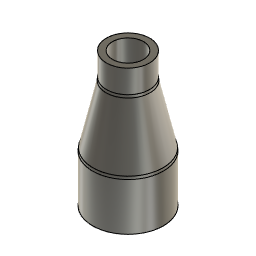
v1.0.0-1.75-to-1.00-reducer (Autodesk Fusion 360 design; units mm, degrees)
Autodesk Fusion 360 part; units mm, degrees
sketch "Sketch12" plane through (0, 0, 0) normal (0, 1, 0) x (1, 0, 0)
  line L0 (92.7232, -0.0199) -> (92.7232, -40.0199)
  line L1 (92.7232, -40.0199) -> (81.4368, -90.0199)
  line L2 (81.4368, -90.0199) -> (81.4368, -110.0199)
  line L3 (81.4368, -110.0199) -> (76.4368, -110.0199)
  line L4 (76.4368, -110.0199) -> (76.4368, -90.0199)
  line L5 (76.4368, -90.0199) -> (87.7232, -40.0199)
  line L6 (87.7232, -40.0199) -> (87.7232, -0.0199)
  line L7 (87.7232, -0.0199) -> (92.7232, -0.0199)
  line L8 (63.7368, -110.603) -> (63.7368, -0.0809)
  dimension "d16" = 5
  dimension "d17" = 5
  dimension "d18" = 50
  dimension "d19" = 20
  dimension "d20" = 40
  dimension "d21" = 12.7
  constraint vertical L0
  constraint parallel L0 L2
  constraint perpendicular L2 L3
  constraint perpendicular L3 L6
  constraint perpendicular L0 L7
  constraint parallel L2 L4
  constraint parallel L1 L5
  constraint equal L2 L4
  constraint vertical L8
  measures "d16" distance of L2.end L3.end
  measures "d17" distance of L0.start L6.end
  measures "d18" vertical distance of L4.end L5.end
  measures "d19" distance of L1.end L2.end
  measures "d20" distance of L0.start L0.end
  measures "d21" distance of L4 L8
revolve "Revolve1" add sketch "Sketch12" angle 360 about axis through (63.7368, 0, 110.603) along (0, 0, -1)
fillet "Fillet1" radius 10 1 edges at (47.2346, -6.4006, 90.0199)
fillet "Fillet2" radius 10 1 edges at (36.7121, -10.4819, 40.0199)
